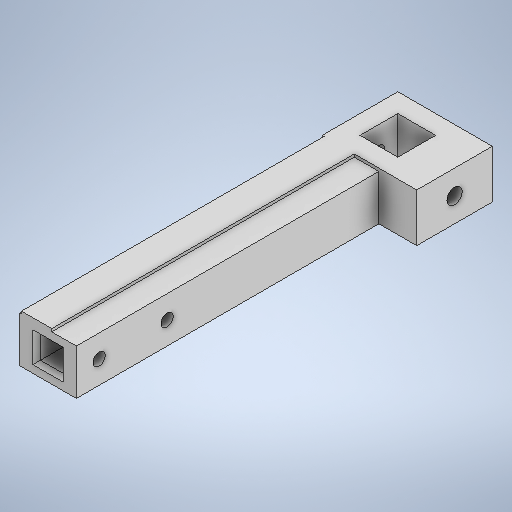
# Autodesk Inventor part: cremaillere
Saved by Autodesk Inventor 2025.2 (Build 292293000, 293)
## iProperties
Created: 2025-03-30
Part Number: cremaillere
Material: Générique
Document SubType Name: Modeling
Designer: enezl
Density: 1 g/cm^3
Appearance: Par défaut
Author: enezl
Autodesk Inventor part; units mm, degrees
ref_plane "YZ Plane" through (0, 0, 0) normal (1, 0, 0) x (0, 1, 0)
ref_plane "XZ Plane" through (0, 0, 0) normal (0, 1, 0) x (-1, 0, 0)
ref_plane "XY Plane" through (0, 0, 0) normal (0, 0, 1) x (1, 0, 0)
sketch "dent" plane through (0, 0, 0) normal (0, 0, 1) x (1, 0, 0)
  line L0 (3.4049, 12.8641) -> (5.6549, 12.0451)
  line L1 (5.6549, 12.0451) -> (5.6549, 11.2941)
  line L2 (5.6549, 11.2941) -> (3.4049, 10.4751)
  line L3 (3.4049, 10.4751) -> (3.4049, 9.7241)
  point P0 (4.4433, 11.2784)
  dimension "d0" = 2.25
  dimension "d1" = 110
  dimension "d2" = 40
  dimension "d3" = 3.14
  measures "d0" distance between parallel lines of L3 L1
  measures "d1" angle of L3 L2
  measures "d2" angle of L2 L0
  measures "d3" distance of L3.end L0.start
sketch "Esquisse1" plane through (0, 0, 0) normal (1, 0, 0) x (0, 1, 0)
  line L0 (12.75, 135) -> (12.75, -15) construction
  line L1 (12.75, 135) -> (2, 135) construction
  line L2 (0, 135) -> (0, -135) construction
  line L3 (0, -135) -> (12.75, -135)
  line L4 (12.75, -15) -> (12.75, -35) construction
  line L5 (2, 135) -> (0, 89.1925) construction
  line L6 (2, 135) -> (0, 135) construction
  line L7 (0, 89.1925) -> (0, -35) construction
  line L8 (12.75, -35) -> (0, -35)
  line L9 (12.75, -35) -> (12.75, -135)
  line L10 (0, -35) -> (0, -135)
  point P0 (0, 0)
  point P1 (0, 0)
  dimension "d4" = 150
  dimension "d13" = 270
  dimension "d14" = 2.5
  dimension "d15" = 2
  dimension "d39" = 170
  dimension "d40" = 12.75
  constraints: 22 end point, 4 perpendicular, 3 vertical, 2 collinear, 2 horizontal, 1 coincident, 1 midpoint, 1 point on line
  measures "d4" distance of L0.start L0.end
  measures "d13" distance of L2.start L2.end
  measures "d14" angle of L2 L5
  measures "d15" distance of L1.end L2.start
  measures "d39" distance between parallel lines of L1 L8
  measures "d40" distance between parallel lines of L4 L2
extrude "Extrusion1" add sketch "Esquisse1" along normal blind 8
sketch "Esquisse2" plane through (8, 0, 0) normal (1, 0, 0) x (0, 0, -1)
  line L0 (135, 0) -> (135, 12.75) projected
  line L1 (115, 12) -> (115, 12.75)
  line L2 (135, 12.75) -> (115, 12.75)
  line L3 (35, 12.75) -> (35, 0) construction
  line L4 (35, 12) -> (35, 0)
  line L5 (35, 12) -> (115, 12)
  line L6 (35, 0) -> (135, 0)
  dimension "d38" = 20
  dimension "d41" = 12
  constraints: 10 end point, 2 horizontal, 2 point on line, 1 collinear, 1 perpendicular, 1 vertical
  measures "d38" distance between parallel lines of L0 L1
  measures "d41" distance between parallel lines of L6 L5
extrude "Extrusion2" add sketch "Esquisse2" along normal blind 6.5 and the other way blind 8.5
sketch "Esquisse3" plane through (14.5, 0, 0) normal (1, 0, 0) x (0, 0, -1)
  line L0 (135, 0) -> (115, 0)
  line L1 (115, 0) -> (115, 12.75)
  line L2 (115, 12.75) -> (135, 12.75)
  line L3 (135, 12.75) -> (135, 0)
  line L4 (125, 12.75) -> (125, 0) construction
  line L5 (135, 12.75) -> (115, 12.75) projected
  point P0 (125, 6.375)
  point P1 (125, 6.375)
  point P2 (125, 6.375)
  dimension "d22" = 20
  constraints: 10 end point, 3 midpoint, 2 coincident, 2 parallel, 1 collinear, 1 horizontal, 1 perpendicular
  measures "d22" distance between parallel lines of L3 L1
extrude "Extrusion3" add sketch "Esquisse3" along normal blind 10
hole "Perçage1" at (14.5, 6.375, -125) direction (-1, 0, 0) diameter 3.2 end through all start extended yes counterbore diameter 4 counterbore depth 2
sketch "Esquisse4" plane through (0, 12.75, 132.6111) normal (0, 1, 0) x (1, 0, 0)
  line L0 (14.5, 252.6111) -> (4.5, 252.6111)
  line L1 (4.5, 252.6111) -> (4.5, 262.6111)
  line L2 (4.5, 262.6111) -> (14.5, 262.6111)
  line L3 (14.5, 262.6111) -> (14.5, 252.6111)
  line L4 (14.5, 252.6111) -> (4.5, 262.6111) construction
  line L5 (4.5, 252.6111) -> (14.5, 262.6111) construction
  line L6 (24.5, 247.6111) -> (24.5, 267.6111) construction
  line L7 (24.5, 257.6111) -> (-0.5, 257.6111) construction
  line L8 (-0.5, 256.0111) -> (-0.5, 259.2111) construction
  point P0 (0, 132.6111)
  point P1 (9.5, 257.6111)
  dimension "d32" = 10
  dimension "d33" = 10
  dimension "d42" = 5
  constraints: 14 end point, 4 midpoint, 2 parallel, 1 horizontal, 1 perpendicular, 1 point on line
  measures "d32" distance of L0.end L1.end
  measures "d33" distance of L1.end L2.end
  measures "d42" distance between parallel lines of L1 L8
extrude "Extrusion4" cut sketch "Esquisse4" against normal through all
sketch "Esquisse5" plane through (0, 12.75, -35) normal (0, 0, 1) x (1, 0, 0)
  line L0 (4, -3.75) -> (10, -3.75)
  line L1 (10, -3.75) -> (10, -9.75)
  line L2 (10, -9.75) -> (4, -9.75)
  line L3 (4, -9.75) -> (4, -3.75)
  line L4 (4, -3.75) -> (10, -9.75) construction
  line L5 (10, -3.75) -> (4, -9.75) construction
  line L6 (14.5, -12.75) -> (14.5, -0.75) construction
  line L7 (14.5, -6.75) -> (-0.5, -6.75) construction
  line L8 (-0.5, -7.975) -> (-0.5, -4.775) construction
  point P0 (0, -12.75)
  point P1 (7, -6.75)
  dimension "d43" = 6
  constraints: 14 end point, 4 midpoint, 2 horizontal, 2 parallel, 2 perpendicular, 1 point on line
  measures "d43" distance of L0.start L0.end
extrude "Extrusion5" cut sketch "Esquisse5" against normal blind 35
chamfer "Chanfrein1" distance 1 angle 45 4 edges at (4, 6, -35) (7, 9, -35) (10, 6, -35) (7, 3, -35)
sketch "Esquisse6" plane through (14.5, 0, 0) normal (1, 0, 0) x (0, 0, -1)
  line L0 (35, 0) -> (35, 12) construction
  line L1 (35, 6) -> (65, 6) construction
  line L2 (41, 6) -> (59, 6) construction
  point P0 (0, 0)
  point P1 (50, 6)
  dimension "d49" = 30
  dimension "d50" = 18
  constraints: 4 end point, 3 midpoint, 2 coincident, 2 point on line, 1 horizontal
  measures "d49" distance of L1.start L1.end
  measures "d50" distance of L2.end L2.start
hole "Perçage2" at (14.5, 6, -41) at (14.5, 6, -59) direction (-1, 0, 0) diameter 2.2 end through all start extended yes counterbore diameter 3.2 counterbore depth 6
